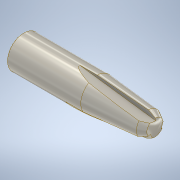
# Autodesk Inventor part: 3.5X13 Implant
Saved by Autodesk Inventor 2022 (Build 260153000, 153)
## iProperties
Created: 2017-05-23
Part Number: 3.5X13 Implant
Material: Titanium
Document SubType Name: Modeling
Designer: SHREEHARI B
Density: 4.51 g/cm^3
Appearance: Titanium - Polished
Mass: 0.226645 g
Surface Area: 2.21859 cm^2
Volume: 0.0502538 cm^3
Sheet Metal Rule: Default
Author: SHREEHARI B
Autodesk Inventor part; units mm, degrees
ref_plane "YZ Plane" through (0, 0, 0) normal (1, 0, 0) x (0, 1, 0)
ref_plane "XZ Plane" through (0, 0, 0) normal (0, 1, 0) x (-1, 0, 0)
ref_plane "XY Plane" through (0, 0, 0) normal (0, 0, 1) x (1, 0, 0)
sketch "Sketch1" plane through (0, 0, 0) normal (0, 1, 0) x (-1, 0, 0)
  line L0 (0, 0) -> (0, 1.6)
  line L1 (0, 1.6) -> (-7.2, 1.6)
  line L2 (-7.2, 1.6) -> (-12.2, 1.1626)
  line L3 (-12.7, 0.8837) -> (-12.7, 0)
  line L4 (-12.7, 0) -> (0, 0)
  line L5 (-12.7, 0) -> (-13, 0)
  line L6 (-12.2, 0) -> (-12.2, 1.1626)
  line L7 (-12.2, 1.1626) -> (-12.85, 0.8)
  line L8 (-12.2, -1.1626) -> (-12.85, -0.8)
  arc A0 (-12.85, 0.8) -> (-12.85, -0.8) centre (-10.7917, 0) ccw
  dimension "d0" = 1.6
  dimension "d1" = 7.2
  dimension "d3" = 12.7
  dimension "d4" = 0.3
  dimension "d352" = 0.8
  dimension "d353" = 0.8
  dimension "d355" = 0.65
  dimension "d359" = 5
  dimension "d373" = 60.848
  constraints: 18 end point, 3 point on circle, 2 perpendicular, 2 point on line, 2 symmetric about line, 2 vertical, 1 centre point, 1 horizontal, 1 parallel
  measures "d0" distance of L0.start L0.end
  measures "d1" distance of L0.end L1.end
  measures "d3" distance between parallel lines of L0 L3
  measures "d4" distance of L3.end L5.end
  measures "d352" distance from line of L5.end L6
  measures "d353" distance from line of L7.end L5
  measures "d355" horizontal distance of L2.end L7.end
  measures "d359" angle of L2 L4
  measures "d373" angle of L6 L7
revolve "Revolution1" add sketch "Sketch1" angle 360 about axis through (12.7, 0, 0) along (-1, 0, 0)
sketch "Sketch2" plane through (0, 0, 0) normal (0, 1, 0) x (-1, 0, 0)
  line L0 (0, -1.35) -> (0, 0)
  line L1 (0, 0) -> (-6.9, 0)
  line L2 (-6.9, 0) -> (-6.9, -0.675)
  line L3 (-6.9, -0.675) -> (-2.8, -0.675)
  line L4 (-2.8, -0.675) -> (-2.8, -1.1)
  line L5 (-2.8, -1.1) -> (-1.35, -1.1)
  line L6 (-1.35, -1.1) -> (-1.35, -1.0753)
  line L7 (-1.35, -1.0753) -> (0, -1.35)
  line L8 (-6.9, -0.675) -> (-7.3619, 0)
  line L9 (-7.3619, 0) -> (-6.9, 0) construction
  line L10 (-7.3619, 0) -> (-6.9, 0)
  line L11 (0, 0) -> (0, -1.425)
  line L12 (0, -1.6) -> (0, 1.6) projected
  line L13 (0, -1.425) -> (0.3686, -1.425)
  dimension "d9" = 1.1
  dimension "d11" = 1.35
  dimension "d12" = 11.5
  dimension "d145" = 0.4619
  dimension "d284" = 1.45
  dimension "d293" = 1.35
  dimension "d361" = 1.425
  dimension "d363" = 0.3686
  dimension "d367" = 6.9
  dimension "d374" = 0.675
  constraints: 26 end point, 6 perpendicular, 2 coincident, 2 point on line, 1 collinear, 1 horizontal, 1 vertical
  measures "d9" distance between parallel lines of L1 L5
  measures "d11" distance of L0.start L0.end
  measures "d12" angle of L1 L7
  measures "d145" distance of L8.end L1.end
  measures "d284" distance of L4.end L5.end
  measures "d293" distance from line of L6.end L0
  measures "d361" distance of L0.end L11.end
  measures "d363" distance of L11.end L13.end
  measures "d367" distance between parallel lines of L2 L12
  measures "d374" distance between parallel lines of L3 L1
revolve "Revolution2" cut sketch "Sketch2" angle 360 about axis through (0, 0, 0) along (1, 0, 0)
sketch "Sketch3" plane through (1.35, 0, 0) normal (1, 0, 0) x (0, 0, -1)
  line L0 (0, 1.299) -> (1.125, 0.6495)
  line L1 (1.125, 0.6495) -> (1.125, -0.6495)
  line L2 (1.125, -0.6495) -> (0, -1.299)
  line L3 (0, -1.299) -> (-1.125, -0.6495)
  line L4 (-1.125, -0.6495) -> (-1.125, 0.6495)
  line L5 (-1.125, 0.6495) -> (0, 1.299)
  point P0 (0, 0)
  point P1 (0, 0)
  dimension "d20" = 0
  dimension "d21" = 2.25
  constraints: 12 end point, 1 coincident, 13 other
  measures "d20" horizontal distance of point (0, 0) L0.start
  measures "d21" distance between parallel lines of L1 L4
extrude "Extrusion1" cut sketch "Sketch3" along normal blind 1.25 and the other way blind 2
fillet "Fillet1" radius 0.05 1 edges at (0, 0, -1.6)
sketch "Sketch10" plane through (0, 0, 0) normal (0, 1, 0) x (-1, 0, 0)
  circle A0 centre (-1.8, 1.5) radius 0.1
  line L0 (-0.5216, -1.4433) -> (-0.46, -1.55)
  line L1 (-0.46, -1.55) -> (-0.6332, -1.55)
  line L2 (-0.6332, -1.55) -> (-0.5716, -1.4433)
  line L3 (-0.5216, -1.4433) -> (-0.5716, -1.4433)
  line L4 (0, 1.55) -> (0, -1.55) projected
  point P0 (0, 0)
  point P1 (-0.5466, -1.5)
  point P2 (-0.5466, -1.4)
  dimension "d69" = 0.2
  dimension "d70" = 1.5
  dimension "d71" = 1.8
  dimension "d232" = 0.15
  dimension "d233" = 0.05
  dimension "d234" = 0.05
  dimension "d235" = 0.46
  dimension "d236" = 1.55
  dimension "d237" = 1.55
  constraints: 8 end point, 2 point on line, 1 centre point, 7 other
  measures "d69" diameter of A0
  measures "d70" vertical distance of point (0, 0) A0.centre
  measures "d71" horizontal distance of point (0, 0) A0.centre
  measures "d232" distance from line of L1 point (-0.547, -1.4)
  measures "d233" distance of L0.start point (-0.547, -1.4)
  measures "d234" distance of L2.end point (-0.547, -1.4)
  measures "d235" distance from line of L4 L0.end
  measures "d236" distance from line of point (0, 0) L1
  measures "d237" vertical distance of L1.end point (0, 0)
sketch "Sketch24" plane through (0, 0, 0) normal (0, 1, 0) x (-1, 0, 0)
  line L0 (-2.0692, 1.4443) -> (-2.5292, 1.4)
  line L1 (-2.5292, 1.4) -> (-3.1116, 2.2165)
  line L2 (-3.1116, 2.2165) -> (-2, 2.3235)
  line L3 (-2, 2.3235) -> (-2.0692, 1.4443)
  line L4 (-2.6, -1.125) -> (-0.2505, -1.125) projected
  line L5 (0, 1.35) -> (0, -1.35) projected
  point P0 (0, 0)
  point P1 (-0.3734, 1.125)
  point P2 (-2.65, 1.125)
  point P3 (-0.2505, -1.125)
  dimension "d167" = 60
  dimension "d170" = 2
  dimension "d171" = 100
  dimension "d357" = 0.8685
  dimension "d358" = 0.46
  dimension "d370" = 1.4
  dimension "d371" = 84.5
  constraints: 9 end point, 1 parallel, 1 other
  measures "d167" angle of L1 L0
  measures "d170" horizontal distance of point (0, 0) L2.end
  measures "d171" angle of L2 L3
  measures "d357" distance between parallel lines of L0 L2
  measures "d358" horizontal distance of L0.start L0.end
  measures "d370" vertical distance of L0.end point (0, 0)
  measures "d371" angle of L0 L5
coil "Coil12" [suppressed]
coil "Coil16" [suppressed]
sketch "Sketch41" plane through (2.0889, 1.4266, -0.4635) normal (0, -0.309, -0.9511) x (1, 0, 0)
  line L0 (0.1155, 0) -> (0.0827, 0.0567) projected
  line L1 (0.0827, 0.0567) -> (0.0327, 0.0567) projected
  line L2 (-0.4173, 0.0567) -> (-0.4673, 0.0567) projected
  line L3 (-0.9173, 0.0567) -> (-0.9673, 0.0567) projected
  line L4 (-1.4173, 0.0567) -> (-1.4673, 0.0567) projected
  line L5 (-1.2173, 2.9433) -> (-1.1673, 2.9433) projected
  line L6 (-0.7173, 2.9433) -> (-0.6673, 2.9433) projected
  line L7 (-0.2173, 2.9433) -> (-0.1673, 2.9433) projected
  arc A0 (-2.0889, 0.05) -> (-2.0389, 0) centre (-2.0389, 0.05) ccw projected
  line L8 (-2.0889, 0.05) -> (-2.0889, 0.15) projected
  line L9 (-2.0889, 0.15) -> (-1.1065, 0.3499) projected
  line L10 (4.8111, 0.7) -> (5.273, 1.5) projected
  line L11 (5.273, 1.5) -> (4.8111, 2.3) projected
  line L12 (-1.1065, 2.6501) -> (-2.0889, 2.85) projected
  line L13 (-2.0889, 2.85) -> (-2.0889, 2.95) projected
  arc A1 (-2.0389, 3) -> (-2.0889, 2.95) centre (-2.0389, 2.95) ccw projected
  line L14 (4.8111, 2.3) -> (0.7111, 2.3) projected
  line L15 (0.7111, 0.7) -> (4.8111, 0.7) projected
  line L16 (0.7111, 2.3) -> (0.7111, 2.6) projected
  line L17 (0.5111, 0.4) -> (0.7111, 0.4) projected
  line L18 (0.7111, 2.6) -> (0.5111, 2.6) projected
  line L19 (0.7111, 0.4) -> (0.7111, 0.7) projected
  line L20 (0, 0) -> (-0.3845, 0) projected
  line L21 (0.0327, 0.0567) -> (0, 0) projected
  line L22 (0.1155, 0) -> (0, 0) projected
  line L23 (0.5111, 0.3499) -> (0.5111, 0.4) projected
  line L24 (0.5111, 2.6) -> (0.5111, 2.6501) projected
  arc A2 (9.2611, 0.6) -> (9.2611, 2.4) centre (6.6361, 1.5) ccw projected
  line L25 (0.5111, 2.6501) -> (-1.1065, 2.6501) projected
  line L26 (4.9111, 0) -> (0.1155, 0) projected
  line L27 (-1.1065, 0.3499) -> (0.5111, 0.3499) projected
  line L28 (9.2611, 0.6) -> (8.6111, 0.3237) projected
  line L29 (8.6111, 0.3237) -> (4.9111, 0) projected
  line L30 (-0.5, 0) -> (-0.8845, 0) projected
  line L31 (-1, 0) -> (-1.3845, 0) projected
  line L32 (-1.5, 0) -> (-2.0389, 0) projected
  line L33 (-2.0389, 3) -> (-1.25, 3) projected
  line L34 (-1.1345, 3) -> (-0.75, 3) projected
  line L35 (-0.6345, 3) -> (-0.25, 3) projected
  line L36 (-0.1345, 3) -> (4.9111, 3) projected
  line L37 (4.9111, 3) -> (8.6111, 2.6763) projected
  line L38 (8.6111, 2.6763) -> (9.2611, 2.4) projected
  point P0 (-2.0889, 1.5)
  point P1 (0.04, 2.55)
  point P2 (0.04, 0.95)
  point P3 (2.4363, -2.336)
  point P4 (2.2646, -2.336)
  point P5 (1.6424, -2.336)
  point P6 (1.4156, -2.336)
  point P7 (0.8485, -2.336)
  point P8 (0.5666, -2.336)
  point P9 (0.14, 0.3317)
  point P10 (0.14, 2.6683)
  point P11 (-0.69, 0)
  point P12 (-0.5168, 0)
  point P13 (-1.15, 0)
  point P14 (0.0554, 3.4951)
  point P15 (0.4369, 3.5)
  point P16 (5.5075, 3.4591)
  point P17 (9.4087, 0.8232)
  point P18 (9.1185, 0.3568)
  point P19 (9.1075, 0.3559)
  point P20 (8.3185, 0.2868)
  point P21 (8.3075, 0.2859)
  point P22 (7.5185, 0.2168)
  point P23 (7.5075, 0.2159)
  point P24 (6.7185, 0.1469)
  point P25 (6.7075, 0.1459)
  point P26 (5.9185, 0.0769)
  point P27 (5.9075, 0.0759)
  point P28 (5.1185, 0.0069)
  point P29 (5.1075, 0.0059)
  point P30 (0, 0.0001)
  point P31 (10.24, 3.1065)
  point P32 (9.9229, 0.3686)
  point P33 (9.8272, 0.361)
  point P34 (9.1222, 0.3055)
  point P35 (9.0317, 0.2984)
  point P36 (8.3215, 0.2425)
  point P37 (8.2362, 0.2358)
  point P38 (7.5207, 0.1795)
  point P39 (7.4407, 0.1732)
  point P40 (6.72, 0.1165)
  point P41 (6.6452, 0.1106)
  point P42 (5.9192, 0.0535)
  point P43 (5.8497, 0.048)
  point P44 (5.1195, 0)
  point P45 (5.0443, 0)
  point P46 (4.2066, 0)
  point P47 (3.5312, 0)
  point P48 (3.3689, 0)
  point P49 (2.7371, 0)
  point P50 (2.5311, 0)
  point P51 (1.943, 0)
  point P52 (1.6934, 0)
  point P53 (1.1489, 0)
  point P54 (0.8557, 0)
  point P55 (10.3292, 3.0438)
  point P56 (10.225, 3.1077)
  point P57 (9.5226, 3.163)
  point P58 (9.4295, 3.1703)
  point P59 (8.7218, 3.226)
  point P60 (8.634, 3.2329)
  point P61 (7.9211, 3.289)
  point P62 (7.8385, 3.2955)
  point P63 (7.1203, 3.352)
  point P64 (7.043, 3.3581)
  point P65 (6.3196, 3.415)
  point P66 (6.2475, 3.4207)
  point P67 (5.5189, 3.4781)
  point P68 (5.4519, 3.4833)
  point P69 (4.7224, 3.5)
  point P70 (4.6255, 3.5)
  point P71 (3.9283, 3.5)
  point P72 (3.7877, 3.5)
  point P73 (3.1342, 3.5)
  point P74 (2.95, 3.5)
  point P75 (2.3401, 3.5)
  point P76 (2.1123, 3.5)
  point P77 (1.5459, 3.5)
  point P78 (1.2745, 3.5)
  point P79 (0.7518, 3.5)
  point P80 (0.4368, 3.5)
  point P81 (0.0559, 3.4961)
  point P82 (-0.0003, 0)
  point P83 (1.2685, 3)
  point P84 (0.6925, 3)
  point P85 (2.1062, 3)
  point P86 (2.9439, 3)
  point P87 (1.4866, 3)
  point P88 (3.7817, 3)
  point P89 (2.2807, 3)
  point P90 (3.0748, 3)
  point P91 (4.6194, 3)
  point P92 (3.8689, 3)
  point P93 (4.6631, 3)
  point P94 (9.3294, 0.7244)
  point P95 (8.9446, 0.4186)
  point P96 (5.4339, 2.9655)
  point P97 (5.461, 2.9636)
  point P98 (6.2339, 2.9095)
  point P99 (6.261, 2.9076)
  point P100 (7.0339, 2.8536)
  point P101 (7.061, 2.8517)
  point P102 (7.8339, 2.7976)
  point P103 (7.861, 2.7957)
  point P104 (8.6339, 2.7417)
  point P105 (8.261, 0.2322)
  point P106 (7.461, 0.1763)
  point P107 (8.2339, 0.2303)
  point P108 (6.661, 0.1203)
  point P109 (7.4339, 0.1744)
  point P110 (5.861, 0.0644)
  point P111 (6.6339, 0.1184)
  point P112 (5.061, 0.0085)
  point P113 (5.8339, 0.0625)
  point P114 (9.0823, 0.491)
  point P115 (-0.7468, 0)
  point P116 (5.0339, 0.0066)
  point P117 (-1.2068, 0)
  point P118 (0.1351, 3)
  point P119 (0.9307, 3)
  point P120 (0.6796, 3)
  point P121 (1.5195, 3)
  point P122 (1.7263, 3)
  point P123 (2.3594, 3)
  point P124 (2.5219, 3)
  point P125 (3.1993, 3)
  point P126 (3.3175, 3)
  point P127 (4.0392, 3)
  point P128 (4.113, 3)
  point P129 (5.6716, 2.9335)
  point P130 (5.7097, 2.9301)
  point P131 (6.4622, 2.8643)
  point P132 (6.5109, 2.86)
  point P133 (7.2527, 2.7951)
  point P134 (7.312, 2.79)
  point P135 (8.0433, 2.726)
  point P136 (8.1131, 2.7199)
  point P137 (8.7927, 2.5991)
  point P138 (8.9225, 2.5439)
  point P139 (9.115, 0.5379)
  point P140 (8.5136, 0.3152)
  point P141 (8.4386, 0.3086)
  point P142 (7.7125, 0.2451)
  point P143 (7.648, 0.2394)
  point P144 (6.9114, 0.175)
  point P145 (6.8574, 0.1703)
  point P146 (6.1103, 0.1049)
  point P147 (6.0669, 0.1011)
  point P148 (5.3092, 0.0348)
  point P149 (5.2763, 0.0319)
  point P150 (4.9086, 3)
  point P151 (4.8791, 3)
  constraints: 16 other
extrude "Extrusion19" [suppressed]
sketch "Sketch45" plane through (0, 0, 0) normal (0, 1, 0) x (-1, 0, 0)
  point P0 (0, 0)
sketch "Sketch47" plane through (0, 0, 0) normal (0, 0, 1) x (1, 0, 0)
  line L0 (0, -1.35) -> (0.2505, -1.299) projected
  line L1 (6.9, -0.675) -> (7.3619, 0) projected
  line L2 (7.3619, 0) -> (6.9, 0.675) projected
  line L3 (0.2505, 1.299) -> (0, 1.35) projected
  line L4 (6.9, 0.675) -> (2.8, 0.675) projected
  line L5 (2.8, -0.675) -> (6.9, -0.675) projected
  arc A0 (0, -1.55) -> (0.05, -1.6) centre (0.05, -1.55) ccw projected
  line L6 (0, -1.55) -> (0, -1.35) projected
  line L7 (0, 1.35) -> (0, 1.55) projected
  arc A1 (0.05, 1.6) -> (0, 1.55) centre (0.05, 1.55) ccw projected
  line L8 (0.2505, -1.299) -> (2.6, -1.299) projected
  line L9 (2.6, -1.299) -> (2.6, -1.1) projected
  line L10 (2.6, 1.1) -> (2.6, 1.299) projected
  line L11 (2.6, 1.299) -> (0.2505, 1.299) projected
  line L12 (2.6, -1.1) -> (2.8, -1.1) projected
  line L13 (2.8, -1.1) -> (2.8, -0.675) projected
  line L14 (2.8, 0.675) -> (2.8, 1.1) projected
  line L15 (2.8, 1.1) -> (2.6, 1.1) projected
  line L16 (12.2, 1.1626) -> (12.85, 0.8) projected
  arc A2 (12.85, -0.8) -> (12.85, 0.8) centre (10.7917, 0) ccw projected
  line L17 (12.85, -0.8) -> (12.2, -1.1626) projected
  line L18 (12.2, -1.1626) -> (7.2, -1.6) projected
  line L19 (7.2, -1.6) -> (0.05, -1.6) projected
  line L20 (0.05, 1.6) -> (7.2, 1.6) projected
  line L21 (7.2, 1.6) -> (12.2, 1.1626) projected
  point P0 (0, 0)
  point P1 (7.012, 0)
sketch "Sketch9" plane through (0, 0, 0) normal (0, 1, 0) x (-1, 0, 0)
  line L0 (0, 1.35) -> (0, -1.35) projected
  line L1 (0, -1.6) -> (0, 1.6) projected
  line L2 (-14.5, 1.6) -> (-5.5, 1.6)
  line L3 (-7.2, 1.6) -> (0, 1.6) projected
  line L4 (-14.5, 1.6) -> (-14.5, 0.4)
  line L5 (-14.5, 0.4) -> (-5.5, 1.6)
  point P0 (0, 0)
  dimension "d257" = 1.2
  dimension "d258" = 5.5
  dimension "d262" = 9
  constraints: 6 end point, 1 collinear, 1 perpendicular, 1 point on line
  measures "d257" distance of L2.start L4.end
  measures "d258" distance of L1.end L2.end
  measures "d262" distance of L2.start L2.end
extrude "Extrusion4" cut sketch "Sketch9" against normal blind 2
pattern_circular "Circular Pattern1" count 3 over 360 about axis through (-10, 0, 0) along (1, 0, 0) of "Extrusion4"
sketch "Sketch50" plane through (0, 0, 0) normal (0, 1, 0) x (-1, 0, 0)
  line L0 (-2.8, 0.675) -> (-6.9, 0.675) projected
  line L1 (-6.9, 0.675) -> (-7.3619, 0) projected
  line L2 (-6.9, -0.675) -> (-2.8, -0.675) projected
  arc A0 (-0.05, -1.6) -> (0, -1.55) centre (-0.05, -1.55) ccw projected
  arc A1 (0, 1.55) -> (-0.05, 1.6) centre (-0.05, 1.55) ccw projected
  line L3 (-0.05, -1.6) -> (-7.2, -1.6) projected
  line L4 (-1.1059, -1.125) -> (0, -1.35) projected
  line L5 (0, -1.35) -> (0, -1.55) projected
  line L6 (0, 1.55) -> (0, 1.35) projected
  line L7 (0, 1.35) -> (-1.1059, 1.125) projected
  line L8 (-2.6, -1.125) -> (-1.1059, -1.125) projected
  line L9 (-1.1059, 1.125) -> (-2.6, 1.125) projected
  line L10 (-2.6, 1.125) -> (-2.6, 1.1) projected
  line L11 (-2.6, -1.1) -> (-2.6, -1.125) projected
  line L12 (-2.8, -0.675) -> (-2.8, -1.1) projected
  line L13 (-2.8, -1.1) -> (-2.6, -1.1) projected
  line L14 (-2.6, 1.1) -> (-2.8, 1.1) projected
  line L15 (-2.8, 1.1) -> (-2.8, 0.675) projected
  line L16 (-7.3619, 0) -> (-6.9, -0.675) projected
  line L17 (-5.5, 1.6) -> (-0.05, 1.6) projected
  line L18 (-12.9136, 0.6115) -> (-5.5, 1.6) projected
  line L19 (-7.2, -1.6) -> (-12.2, -1.1626) projected
  line L20 (-12.85, 0.8) -> (-12.2, 1.1626) projected
  line L21 (-12.2, 1.1626) -> (-7.2, 1.6) projected
  line L22 (-7.2, 1.6) -> (-5.5, 1.6) projected
  line L23 (-12.2, -1.1626) -> (-12.85, -0.8) projected
  arc A2 (-12.9136, 0.6115) -> (-12.85, -0.8) centre (-10.7917, 0) ccw projected
  arc A3 (-12.85, 0.8) -> (-12.9136, 0.6115) centre (-10.7917, 0) ccw projected
  point P0 (0, 0)
  point P1 (-1.4382, 1.75)
  point P2 (-1.495, 1.75)
  point P3 (-1.6682, 1.75)
  point P4 (-6.2041, 1.75)
  point P5 (-11.5804, 0.9405)
  point P6 (-2.2986, 1.75)
  point P7 (-5.8766, -1.75)
  point P8 (-6.6717, -1.75)
  point P9 (-7.4687, -1.7289)
  point P10 (-10.5666, -1.2193)
  point P11 (-10.7, -0.8888)
  point P12 (-3.5, -1.3923)
  point P13 (-4.3, -1.3364)
  point P14 (-5.1, -1.2804)
  point P15 (-5.9, -1.2245)
  point P16 (-6.7, -1.1685)
  point P17 (-7.5, -1.1126)
  point P18 (-2.3, 1.4762)
  point P19 (-3.1, 1.4203)
  point P20 (-3.9, 1.3643)
  point P21 (-4.7, 1.3084)
  point P22 (-5.5, 1.2524)
  point P23 (-6.3, 1.1965)
  point P24 (-7.1, 1.1406)
  point P25 (-7.9, 1.0846)
  point P26 (-8.7, 1.0287)
  point P27 (-6.2532, 1.5)
  point P28 (-3.5, -1.3923)
  point P29 (-7.4513, -1.4231)
  point P30 (-8.2513, -1.3601)
  point P31 (-9.0513, -1.2971)
  point P32 (-8.3929, 1.3781)
  constraints: 4 other
sketch "Sketch51" plane through (0, 0, 0) normal (0, 0, 1) x (1, 0, 0)
  line L0 (0, -1.35) -> (0.2505, -1.299) projected
  line L1 (6.9, -0.675) -> (7.3619, 0) projected
  line L2 (7.3619, 0) -> (6.9, 0.675) projected
  line L3 (0.2505, 1.299) -> (0, 1.35) projected
  line L4 (0.05, 1.6) -> (7.1077, 1.6) projected
  line L5 (0, 1.35) -> (0, 1.55) projected
  arc A0 (0.05, 1.6) -> (0, 1.55) centre (0.05, 1.55) ccw projected
  arc A1 (0, -1.55) -> (0.05, -1.6) centre (0.05, -1.55) ccw projected
  line L6 (0, -1.55) -> (0, -1.35) projected
  line L7 (7.2, -1.6) -> (0.05, -1.6) projected
  line L8 (2.6, 1.299) -> (0.2505, 1.299) projected
  line L9 (0.2505, -1.299) -> (2.6, -1.299) projected
  line L10 (2.6, -1.299) -> (2.6, -1.1) projected
  line L11 (2.6, 1.1) -> (2.6, 1.299) projected
  line L12 (6.9, 0.675) -> (2.8, 0.675) projected
  line L13 (2.8, 0.675) -> (2.8, 1.1) projected
  line L14 (2.8, 1.1) -> (2.6, 1.1) projected
  line L15 (2.6, -1.1) -> (2.8, -1.1) projected
  line L16 (2.8, -1.1) -> (2.8, -0.675) projected
  line L17 (2.8, -0.675) -> (6.9, -0.675) projected
  line L18 (12.85, -0.8) -> (12.2, -1.1626) projected
  line L19 (12.2, -1.1626) -> (7.2, -1.6) projected
  line L20 (7.1077, 1.6) -> (12.8824, 0.7109) projected
  arc A2 (12.85, -0.8) -> (12.8824, 0.7109) centre (10.7917, 0) ccw projected
  point P0 (0, 0)
  point P1 (7.012, 0)
  point P2 (0.7475, 1.75)
  point P3 (0.9775, 1.75)
  point P4 (1.2075, 1.75)
  point P5 (8.1591, 1.2076)
  point P6 (5.2803, 1.75)
  point P7 (6.0754, 1.75)
  point P8 (7.6761, 1.6296)
  point P9 (8.4815, 1.5119)
  point P10 (6.0591, 1.5)
  point P11 (10.1597, -0.9266)
  point P12 (9.6652, -1.2902)
  point P13 (8.8644, -1.3533)
  point P14 (7.2629, -1.4793)
  point P15 (9.3597, -0.9825)
  point P16 (3.3597, 1.4021)
  point P17 (4.1597, 1.3462)
  point P18 (6.5597, 1.1783)
  point P19 (7.3597, 1.1224)
  point P20 (8.1597, 1.0665)
  point P21 (9.7597, 0.9546)
  point P22 (10.5597, 0.8986)
  point P23 (10.9597, -0.8707)
  point P24 (8.5597, -1.0385)
  point P25 (7.7597, -1.0944)
  point P26 (6.9597, -1.1504)
  point P27 (5.3597, -1.2622)
  point P28 (4.5597, -1.3182)
  point P29 (3.7597, -1.3741)
  point P30 (2.9597, -1.4301)
  point P31 (3.3597, 1.4021)
  point P32 (9.6652, -1.2902)
  point P33 (10.5597, 0.8986)
  point P34 (8.9597, 0.8491)
  point P35 (10.5597, 0.7232)
  point P36 (6.5597, 1.038)
  point P37 (2.8826, 1.5)
  point P38 (3.6767, 1.5)
  point P39 (4.4708, 1.5)
  point P40 (5.2498, -1.5)
  point P41 (4.0738, -1.5)
  point P42 (3.2796, -1.5)
  constraints: 1 other
sketch "Sketch52" plane through (2.65, 0, 0) normal (-1, 0, 0) x (0, 0, 1)
  circle A0 centre (0, 0) radius 1.125
  dimension "d321" = 2.25
  constraints: 1 centre point, 1 coincident
  measures "d321" diameter of A0
extrude "Extrusion21" [suppressed]
sketch "Sketch53" plane through (0, 0, 0) normal (0, 0, 1) x (1, 0, 0)
  line L0 (2.8, -0.75) -> (3.0165, -0.75)
  line L1 (2.8, -0.75) -> (2.8, -1.125)
  line L2 (2.8, -1.125) -> (3.0165, -0.75)
  line L3 (-2.6183, 0) -> (15.6376, 0) projected
  point P0 (0, 0)
  dimension "d325" = 1.125
  dimension "d326" = 0.75
  dimension "d327" = 60
  dimension "d328" = 2.8
  constraints: 6 end point, 1 horizontal, 1 vertical
  measures "d325" vertical distance of point (0, 0) L1.end
  measures "d326" distance from line of point (0, 0) L0
  measures "d327" angle of L0 L2
  measures "d328" horizontal distance of point (0, 0) L0.start
revolve "Revolution7" [suppressed]
thread "Thread3" size "M1.6x0.35" class "6H" standard "ANSI Metric M Profile" length 3.1
sketch "Sketch54" plane through (0, 0, 0) normal (0, 1, 0) x (-1, 0, 0)
  line L0 (-13, 1.19) -> (-13, 0.25)
  line L1 (2.6183, 0) -> (-15.6376, 0) projected
  line L2 (0, 1.35) -> (0, -1.35) projected
  line L3 (-13, 0.25) -> (-12.6579, 1.19)
  line L4 (-12.6579, 1.19) -> (-13, 1.19)
  point P0 (0, 0)
  point P1 (-12.861, 0.9532)
  dimension "d341" = 13
  dimension "d342" = 0.94
  dimension "d343" = 20
  dimension "d344" = 0.25
  constraints: 6 end point, 1 horizontal
  measures "d341" distance between parallel lines of L2 L0
  measures "d342" distance of L0.start L0.end
  measures "d343" angle of L3 L0
  measures "d344" distance from line of L1 L0.end
revolve "Revolution8" [suppressed]
sketch "Sketch55" plane through (0.5216, 0, -1.4433) normal (0, 1, 0) x (1, 0, 0)
  line L0 (0.05, 0) -> (0.0827, 0.0567) projected
  line L1 (-0.0327, 0.0567) -> (0.0827, 0.0567) projected
  line L2 (-0.4716, 0.0567) -> (-0.0327, 0.0567) projected
  arc A0 (-0.4716, 0.0567) -> (-0.5216, 0.0067) centre (-0.4716, 0.0067) ccw projected
  line L3 (-0.5216, -0.0933) -> (-0.5216, 0.0067) projected
  line L4 (0.5843, -0.3183) -> (-0.5216, -0.0933) projected
  line L5 (6.3784, -0.6433) -> (2.2784, -0.6433) projected
  line L6 (6.8403, -1.4433) -> (6.3784, -0.6433) projected
  line L7 (6.3784, -2.2433) -> (6.8403, -1.4433) projected
  line L8 (2.2784, -2.2433) -> (6.3784, -2.2433) projected
  line L9 (-0.5216, -2.7933) -> (0.5843, -2.5683) projected
  line L10 (-0.5216, -2.8933) -> (-0.5216, -2.7933) projected
  arc A1 (-0.5216, -2.8933) -> (-0.4716, -2.9433) centre (-0.4716, -2.8933) ccw projected
  line L11 (0.5, 0) -> (0.55, 0) projected
  line L12 (1, 0) -> (1.05, 0) projected
  line L13 (1.5, 0) -> (1.55, 0) projected
  line L14 (1.3, -2.8866) -> (1.25, -2.8866) projected
  line L15 (0.8, -2.8866) -> (0.75, -2.8866) projected
  line L16 (0.3, -2.8866) -> (0.25, -2.8866) projected
  line L17 (0, 0) -> (0.05, 0) projected
  line L18 (-0.0327, 0.0567) -> (0, 0) projected
  line L19 (0.0827, 0.0567) -> (0.4673, 0.0567) projected
  line L20 (10.9407, -1.899) -> (3.9784, -2.9433) projected
  line L21 (0.5827, 0.0567) -> (0.9673, 0.0567) projected
  line L22 (1.0827, 0.0567) -> (1.4673, 0.0567) projected
  line L23 (1.5827, 0.0567) -> (6.4784, 0.0567) projected
  line L24 (0.2173, -2.9433) -> (-0.4716, -2.9433) projected
  line L25 (2.2784, -0.6433) -> (2.2784, -0.3433) projected
  line L26 (2.2784, -0.3433) -> (2.0784, -0.3433) projected
  line L27 (2.0784, -0.3433) -> (2.0784, -0.3183) projected
  line L28 (2.0784, -0.3183) -> (0.5843, -0.3183) projected
  line L29 (0.5843, -2.5683) -> (2.0784, -2.5683) projected
  line L30 (2.0784, -2.5683) -> (2.0784, -2.5433) projected
  line L31 (2.0784, -2.5433) -> (2.2784, -2.5433) projected
  line L32 (2.2784, -2.5433) -> (2.2784, -2.2433) projected
  line L33 (3.9784, -2.9433) -> (1.3327, -2.9433) projected
  line L34 (1.2173, -2.9433) -> (0.8327, -2.9433) projected
  line L35 (0.7173, -2.9433) -> (0.3327, -2.9433) projected
  line L36 (6.4784, 0.0567) -> (10.0076, -0.2521) projected
  line L37 (10.0076, -0.2521) -> (10.4686, -0.3904) projected
  line L38 (10.4686, -0.3904) -> (10.8284, -0.5433) projected
  arc A2 (10.9407, -1.899) -> (10.8284, -0.5433) centre (8.2034, -1.4433) ccw projected
  arc A3 (10.8284, -2.3433) -> (10.9407, -1.899) centre (8.2034, -1.4433) ccw projected
  line L39 (10.8284, -2.3433) -> (10.1784, -2.6196) projected
  line L40 (10.1784, -2.6196) -> (6.4784, -2.9433) projected
  line L41 (6.4784, -2.9433) -> (3.9784, -2.9433) projected
  point P0 (-0.5216, -1.4433)
  point P1 (0.2266, -3.3933)
  point P2 (0.4566, -3.3933)
  point P3 (0.6866, -3.3933)
  point P4 (0.9166, -3.3933)
  point P5 (1.1466, -3.3933)
  point P6 (1.3766, -3.3933)
  point P7 (5.6825, -3.3933)
  point P8 (0.3416, 0.1067)
  point P9 (0.5716, 0.1067)
  point P10 (11.0588, -2.5838)
  point P11 (1.6066, -3.3933)
  point P12 (6.4725, -3.3933)
  point P13 (5.7316, -2.8933)
  point P14 (8.1784, -2.422)
  point P15 (10.6381, -0.5366)
  point P16 (2.9784, -0.001)
  point P17 (9.3784, -0.6222)
  point P18 (7.7297, -0.0332)
  point P19 (8.5297, -0.0962)
  point P20 (7.8713, -2.7714)
  point P21 (6.2784, -2.8933)
  constraints: 12 other
extrude "Extrusion22" [suppressed]
sketch "Sketch56" plane through (2.0454, -0.6215, 0.2019) normal (0, -0.309, -0.9511) x (1, 0, 0)
  line L0 (-1.1738, 0.7898) -> (-1.1238, 0.7898) projected
  arc A0 (-1.9954, 0.8465) -> (-2.0454, 0.7965) centre (-1.9954, 0.7965) ccw projected
  line L1 (-2.0454, 0.6965) -> (-2.0454, 0.7965) projected
  line L2 (-1.063, 0.4967) -> (-2.0454, 0.6965) projected
  line L3 (4.8546, -1.4535) -> (5.3165, -0.6535) projected
  line L4 (5.3165, -0.6535) -> (4.8546, 0.1465) projected
  line L5 (-2.0454, -2.0035) -> (-1.063, -1.8036) projected
  line L6 (-2.0454, -2.1035) -> (-2.0454, -2.0035) projected
  arc A1 (-2.0454, -2.1035) -> (-1.9954, -2.1535) centre (-1.9954, -2.1035) ccw projected
  line L7 (-0.6738, 0.7898) -> (-0.6238, 0.7898) projected
  line L8 (-0.1738, 0.7898) -> (-0.1238, 0.7898) projected
  line L9 (-0.3738, -2.0968) -> (-0.4238, -2.0968) projected
  line L10 (-0.8738, -2.0968) -> (-0.9238, -2.0968) projected
  line L11 (-1.3738, -2.0968) -> (-1.4238, -2.0968) projected
  line L12 (0.159, -2.1535) -> (0.1262, -2.0968) projected
  line L13 (0.1262, -2.0968) -> (0.0762, -2.0968) projected
  line L14 (-0.091, 0.8465) -> (0.1785, 0.8465) projected
  line L15 (0.0435, -2.1535) -> (-0.341, -2.1535) projected
  line L16 (0.0762, -2.0968) -> (0.0435, -2.1535) projected
  line L17 (0.159, -2.1535) -> (0.0435, -2.1535) projected
  line L18 (0.5763, -2.1535) -> (0.159, -2.1535) projected
  line L19 (-1.4565, -2.1535) -> (-1.9954, -2.1535) projected
  line L20 (0.7546, -1.4535) -> (4.8546, -1.4535) projected
  line L21 (0.7546, 0.1465) -> (0.7546, 0.4465) projected
  line L22 (0.7546, 0.4465) -> (0.5546, 0.4465) projected
  line L23 (0.5546, 0.4465) -> (0.5546, 0.4967) projected
  line L24 (-1.9954, 0.8465) -> (-1.2065, 0.8465) projected
  line L25 (-1.091, 0.8465) -> (-0.7065, 0.8465) projected
  line L26 (-0.591, 0.8465) -> (-0.2065, 0.8465) projected
  line L27 (0.5546, -1.8036) -> (0.5546, -1.7535) projected
  line L28 (0.5546, -1.7535) -> (0.7546, -1.7535) projected
  line L29 (0.7546, -1.7535) -> (0.7546, -1.4535) projected
  line L30 (4.8546, 0.1465) -> (0.7546, 0.1465) projected
  line L31 (0.7231, 0.8465) -> (0.9741, 0.8465) projected
  line L32 (1.563, 0.8465) -> (1.7697, 0.8465) projected
  line L33 (2.4029, 0.8465) -> (2.5653, 0.8465) projected
  line L34 (3.2428, 0.8465) -> (3.3609, 0.8465) projected
  line L35 (4.0827, 0.8465) -> (4.1565, 0.8465) projected
  line L36 (2.1675, -2.1535) -> (1.983, -2.1535) projected
  line L37 (1.3719, -2.1535) -> (1.1431, -2.1535) projected
  line L38 (0.5546, 0.4967) -> (-1.063, 0.4967) projected
  line L39 (4.9226, 0.8465) -> (4.9521, 0.8465) projected
  line L40 (5.7151, 0.78) -> (5.7532, 0.7767) projected
  line L41 (6.5056, 0.7108) -> (6.5543, 0.7066) projected
  line L42 (7.2962, 0.6417) -> (7.3555, 0.6365) projected
  line L43 (8.0868, 0.5725) -> (8.1566, 0.5664) projected
  line L44 (8.8362, 0.4456) -> (8.966, 0.3905) projected
  arc A2 (9.4152, -1.1196) -> (9.3418, 0.1298) centre (6.6796, -0.6535) ccw projected
  line L45 (9.4152, -1.1196) -> (5.6437, -1.6979) projected
  line L46 (5.3826, -1.738) -> (5.0794, -1.7845) projected
  line L47 (4.5773, -1.8615) -> (4.3223, -1.9006) projected
  line L48 (3.772, -1.985) -> (3.5652, -2.0167) projected
  line L49 (2.9667, -2.1084) -> (2.8081, -2.1328) projected
  line L50 (-0.4565, -2.1535) -> (-0.841, -2.1535) projected
  line L51 (-0.9565, -2.1535) -> (-1.341, -2.1535) projected
  line L52 (-1.063, -1.8036) -> (0.5546, -1.8036) projected
  point P0 (-2.0454, -0.6535)
  point P1 (0.3989, 3.4635)
  point P2 (7.9, 3.2589)
  point P3 (2.9371, 3.5)
  point P4 (0.038, 3.4961)
  point P5 (8.3992, 2.4114)
  point P6 (-0.0008, 0.0012)
  point P7 (3.1992, 0.225)
  point P8 (7.465, 0.5622)
  point P9 (6.6601, 0.4594)
  point P10 (5.8552, 0.3565)
  point P11 (5.0502, 0.2537)
  point P12 (4.8225, 0.3444)
  point P13 (7.4574, 0.5612)
  point P14 (6.6533, 0.4585)
  point P15 (5.8491, 0.3557)
  point P16 (5.0449, 0.253)
  point P17 (5.4232, 2.9217)
  point P18 (6.2232, 2.8587)
  point P19 (7.0232, 2.7958)
  point P20 (8.6232, 2.6699)
  point P21 (5.4232, 2.9217)
  point P22 (0.1838, 0.7796)
  point P23 (0.9838, 0.7237)
  point P24 (0.6438, 0.7354)
  point P25 (1.4438, 0.6794)
  point P26 (1.7838, 0.6678)
  point P27 (2.2438, 0.6235)
  point P28 (2.5838, 0.6118)
  point P29 (3.0438, 0.5675)
  point P30 (3.3838, 0.5559)
  point P31 (3.8438, 0.5116)
  point P32 (4.1838, 0.4999)
  point P33 (4.6438, 0.4556)
  point P34 (4.9838, 0.444)
  point P35 (5.7838, 0.3881)
  point P36 (6.5838, 0.3321)
  point P37 (7.3838, 0.2762)
  point P38 (8.1838, 0.2202)
  point P39 (8.9838, 0.1643)
  point P40 (5.3838, -1.7229)
  point P41 (4.5838, -1.7789)
  point P42 (3.7838, -1.8348)
  point P43 (5.4438, 0.3997)
  point P44 (2.9838, -1.8908)
  point P45 (5.0438, -1.7346)
  point P46 (2.1838, -1.9467)
  point P47 (4.2438, -1.7905)
  point P48 (1.3838, -2.0027)
  point P49 (3.4438, -1.8465)
  point P50 (0.5838, -2.0586)
  point P51 (2.6438, -1.9024)
  point P52 (1.8438, -1.9584)
  point P53 (6.2438, 0.3438)
  point P54 (7.0438, 0.2878)
  point P55 (7.8438, 0.2319)
  point P56 (8.6438, 0.1759)
  point P57 (1.0438, -2.0143)
  constraints: 67 other
extrude "Extrusion23" [suppressed]
sketch "Sketch57" plane through (0.2505, -0.6495, 1.125) normal (0, 0, -1) x (-1, 0, 0)
  point P0 (0.2505, 0.6495)
sketch "Sketch58" plane through (2.1282, 0, 1.5) normal (0, -1, 0) x (1, 0, 0)
  line L0 (-0.0634, 0) -> (0.4723, 0) projected
  line L1 (-4.5095, -1.5) -> (12.087, -1.5) projected
  line L2 (-0.0426, -0.0738) -> (-0.0426, 0)
  line L3 (-0.0426, 0) -> (0, 0)
  line L4 (0.401, -0.1) -> (-0.059, -0.0557) projected
  line L5 (0.4723, 0) -> (0.401, -0.1) projected
  line L6 (-0.059, -0.0557) -> (-0.0634, 0) projected
  point P0 (-2.1282, -1.5)
  constraints: 4 end point, 1 perpendicular, 1 vertical
revolve "Revolution9" [suppressed]
thread "Thread5" size "M1.6x0.35" class "6H" standard "ANSI Metric M Profile" length 3
sketch "Sketch59" plane through (2.0648, 0, 1.5) normal (0, -1, 0) x (1, 0, 0)
  line L0 (0, 0) -> (0.5357, 0) projected
  line L1 (0.0044, -0.0557) -> (0, 0) projected
  line L2 (0.4644, -0.1) -> (0.0044, -0.0557) projected
  line L3 (0.5357, 0) -> (0.4644, -0.1) projected
  line L4 (-4.7473, -1.5) -> (13.9575, -1.5) projected
  point P0 (-2.0648, -1.5)
revolve "Revolution10" [suppressed]
chamfer "Chamfer5" distance 0.2 angle 45 1 edges at (2.8, 0, 0.675)
body "Solid1"
